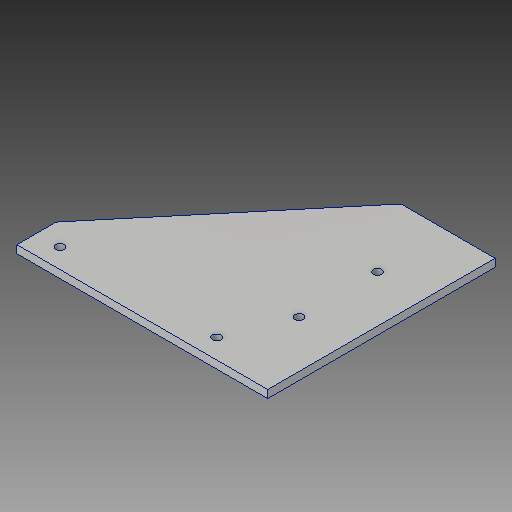
# Autodesk Inventor part: Front Brace
Saved by Autodesk Inventor 2019.4 (Build 234330000, 330)
## iProperties
Created: 2020-01-06
Part Number: Front Brace
Material: Aluminum 6061
Document SubType Name: Modeling
Designer: Mark
Mass: 232.2 g
Surface Area: 371.31 cm^2
Volume: 86 cm^3
Density: 2.7 g/cm^3
Appearance: Aluminum - Flat
Author: Mark
Autodesk Inventor part; units mm, degrees
ref_plane "YZ Plane" through (0, 0, 0) normal (1, 0, 0) x (0, 1, 0)
ref_plane "XZ Plane" through (0, 0, 0) normal (0, 1, 0) x (-1, 0, 0)
ref_plane "XY Plane" through (0, 0, 0) normal (0, 0, 1) x (1, 0, 0)
sketch "Sketch1" plane through (0, 0, 0) normal (0, 1, 0) x (-1, 0, 0)
  line L0 (0, 0) -> (160, 0)
  line L1 (160, 0) -> (160, -145)
  line L2 (160, -145) -> (0, -145)
  line L3 (0, -145) -> (0, 0)
  line L4 (160, 0) -> (0, 0)
  line L5 (0, 0) -> (0, -25)
  line L6 (0, -25) -> (160, -25)
  line L7 (160, -25) -> (160, 0)
  line L8 (0, -145) -> (60, -145)
  line L9 (60, -145) -> (60, -25)
  line L10 (60, -25) -> (0, -25)
  line L11 (0, -25) -> (0, -145)
  line L12 (60, -145) -> (160, -25)
  dimension "d0" = 160
  dimension "d1" = 145
  dimension "d2" = 25
  dimension "d3" = 60
  constraints: 26 end point, 6 parallel, 3 horizontal, 3 perpendicular, 2 point on line
  measures "d0" distance of L1.end L2.end
  measures "d1" distance of L0.end L1.end
  measures "d2" distance of L5.end L4.end
  measures "d3" distance of L10.end L9.end
extrude "Extrusion1" add sketch "Sketch1" along normal blind 5 contours L0 L1 L6 L3 | L6 L9 L2 L3 | L12 L9 L6
fillet "Fillet1" radius 2 2 edges at (-60, 2.5, -145) (-160, 2.5, -25)
sketch "Sketch2" plane through (0, 5, 0) normal (0, 1, 0) x (1, 0, 0)
  circle A0 centre (-30, 50) radius 2.75
  circle A1 centre (-30, 100) radius 2.75
  line L0 (0, 0) -> (0, 145) projected
  line L1 (-160, 0) -> (0, 0) projected
  circle A2 centre (-45, 12.5) radius 2.75
  circle A3 centre (-145, 12.5) radius 2.75
  dimension "d7" = 5.5
  dimension "d8" = 5.5
  dimension "d9" = 30
  dimension "d10" = 30
  dimension "d11" = 50
  dimension "d12" = 50
  dimension "d13" = 5.5
  dimension "d14" = 12.5
  dimension "d15" = 45
  dimension "d16" = 5.5
  dimension "d17" = 100
  dimension "d18" = 12.5
  constraints: 4 centre point
  measures "d7" diameter of A0
  measures "d8" diameter of A1
  measures "d9" distance from line of L0 A0.centre
  measures "d10" distance from line of L0 A1.centre
  measures "d11" distance of A1.centre A0.centre
  measures "d12" distance from line of L1 A0.centre
  measures "d13" diameter of A2
  measures "d14" distance from line of L1 A2.centre
  measures "d15" distance from line of L0 A2.centre
  measures "d16" diameter of A3
  measures "d17" distance of A2.centre A3.centre
  measures "d18" distance from line of L1 A3.centre
extrude "Extrusion2" cut sketch "Sketch2" against normal blind 5
body "Solid1"
